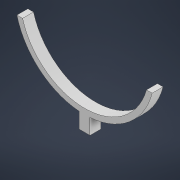
# Autodesk Inventor part: Clip_TestFitV1
Saved by Autodesk Inventor 2022 (Build 260153000, 153)
## iProperties
Created: 2023-05-05
Part Number: Clip_TestFitV1
Material: Generic
Document SubType Name: Modeling
Designer: User
Density: 1 g/cm^3
Appearance: Default
Author: User
Autodesk Inventor part; units mm, degrees
ref_plane "YZ Plane" through (0, 0, 0) normal (1, 0, 0) x (0, 1, 0)
ref_plane "XZ Plane" through (0, 0, 0) normal (0, 1, 0) x (-1, 0, 0)
ref_plane "XY Plane" through (0, 0, 0) normal (0, 0, 1) x (1, 0, 0)
sketch "Sketch1" plane through (0, 0, 0) normal (0, 0, 1) x (1, 0, 0)
  arc A0 (-25.4018, -15) -> (25.4018, -15) centre (0, 0) ccw
  line L0 (2.5, -32) -> (2.5, -39)
  line L1 (2.5, -39) -> (-2.5, -39)
  line L2 (-2.5, -39) -> (-2.5, -32)
  line L3 (-2.5, -32) -> (-2.5, -31.9022)
  line L4 (2.5, -32) -> (2.5, -31.9022)
  arc A1 (-28.2666, -15) -> (-2.5, -31.9022) centre (0, 0) ccw
  arc A2 (2.5, -31.9022) -> (28.2666, -15) centre (0, 0) ccw
  arc A3 (-27.7534, -10) -> (27.7534, -10) centre (0, 0) ccw
  arc A4 (-30.3974, -10) -> (-2.5, -31.9022) centre (0, 0) ccw
  arc A5 (2.5, -31.9022) -> (30.3974, -10) centre (0, 0) ccw
  arc A6 (-28.3945, -8) -> (28.3945, -8) centre (0, 0) ccw
  line L5 (-28.3945, -8) -> (-30.9839, -8)
  line L6 (28.3945, -8) -> (30.9839, -8)
  arc A7 (-30.9839, -8) -> (-2.5, -31.9022) centre (0, 0) ccw
  arc A8 (2.5, -31.9022) -> (30.9839, -8) centre (0, 0) ccw
  point P0 (25.4018, -15)
  point P1 (-28.2666, -15)
  point P2 (27.7534, -10)
  point P3 (-30.3974, -10)
  dimension "d43" = 5
  dimension "d64" = 7
  constraints: 18 point on circle, 14 end point, 9 centre point, 5 coincident, 2 vertical, 1 concentric, 1 parallel
  measures "d43" distance of L0.end L1.end
  measures "d64" distance of L0.start L0.end
extrude "Extrusion7" add sketch "Sketch1" along normal blind 5
body "Solid5"
